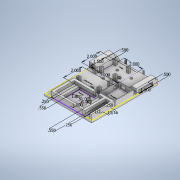
# Autodesk Inventor part: chassis
Saved by Autodesk Inventor 2022 (Build 260153000, 153)
## iProperties
Created: 2021-04-16
Part Number: chassis
Material: Generic
Document SubType Name: Modeling
Designer: kevin
Density: 1 g/cm^3
Appearance: Default
Author: kevin
Autodesk Inventor part; units mm, degrees
ref_plane "YZ Plane" through (0, 0, 0) normal (1, 0, 0) x (0, 1, 0)
ref_plane "XZ Plane" through (0, 0, 0) normal (0, 1, 0) x (-1, 0, 0)
ref_plane "XY Plane" through (0, 0, 0) normal (0, 0, 1) x (1, 0, 0)
sketch "Sketch1" plane through (0, 0, 0) normal (0, 1, 0) x (-1, 0, 0)
  line L0 (63.5, 88.9) -> (-63.5, 88.9)
  line L1 (-63.5, 88.9) -> (-63.5, -88.9)
  line L2 (-63.5, -88.9) -> (63.5, -88.9)
  line L3 (63.5, -88.9) -> (63.5, 88.9)
  line L4 (63.5, 88.9) -> (-63.5, -88.9) construction
  line L5 (-63.5, 88.9) -> (63.5, -88.9) construction
  point P0 (0, 0)
  dimension "d0" = 177.8
  dimension "d1" = 127
  constraints: 12 end point, 2 midpoint, 2 parallel, 1 horizontal, 1 perpendicular
  measures "d0" distance of L2.end L0.start
  measures "d1" distance of L0.start L0.end
extrude "main chassis frame" add sketch "Sketch1" along normal blind 6.35
fillet "chassis front fillet" [suppressed]
fillet "chassis back fillet" [suppressed]
sketch "Sketch3" plane through (63.5, 6.35, 88.9) normal (1, 0, 0) x (0, 0, -1)
  line L0 (0, -6.35) -> (177.8, -6.35) projected
  line L1 (151.8606, -6.35) -> (113.7606, -6.35)
  line L2 (113.7606, -6.35) -> (113.7606, -44.45)
  line L3 (113.7606, -44.45) -> (151.8606, -44.45)
  line L4 (151.8606, -44.45) -> (151.8606, -6.35)
  point P0 (88.9, -6.35)
  point P1 (3.175, -6.35)
  point P2 (174.625, -6.35)
  dimension "d10" = 38.1
  dimension "d11" = 38.1
  constraints: 8 end point, 2 parallel, 1 horizontal, 1 perpendicular, 1 point on line
  measures "d10" distance of L2.end L3.end
  measures "d11" distance of L3.end L1.start
extrude "motor mount" [suppressed]
fillet "round motor mounts" [suppressed]
sketch "Sketch4" plane through (0, 6.35, 0) normal (0, 1, 0) x (1, 0, 0)
  circle A0 centre (15.0812, -75.521) radius 2.3812
  line L0 (15.0812, -75.521) -> (0, -75.521) construction
  circle A1 centre (15.0812, -51.7085) radius 2.3812
  line L1 (15.0812, -51.7085) -> (15.0812, -75.521) construction
  point P0 (0, 0)
  dimension "d15" = 4.7625
  dimension "d17" = 15.0813
  dimension "d19" = 4.7625
  dimension "d20" = 23.8125
  constraints: 4 end point, 2 centre point, 1 horizontal, 1 vertical
  measures "d15" diameter of A0
  measures "d17" distance of L0.start L0.end
  measures "d19" diameter of A1
  measures "d20" distance of L1.start L0.start
extrude "mounting holes for caster" cut sketch "Sketch4" against normal blind 6.35
sketch "Sketch5" plane through (0, 6.35, 0) normal (0, 1, 0) x (1, 0, 0)
  line L0 (63.5, 88.9) -> (-63.5, 88.9) projected
  line L1 (-63.5, -88.9) -> (63.5, -88.9) projected
  line L2 (0, 88.9) -> (-63.5, 88.9)
  line L3 (-63.5, 88.9) -> (-63.5, -88.9)
  line L4 (-63.5, -88.9) -> (0, -88.9)
  line L5 (0, -88.9) -> (0, 88.9)
  point P0 (0, 0)
  point P1 (-63.5, 88.9)
  constraints: 8 end point, 2 parallel, 1 horizontal, 1 midpoint, 1 perpendicular
extrude "cut in half to mirror holes later" cut sketch "Sketch5" against normal blind 6.35
sketch "Sketch6" plane through (0, 0, 0) normal (0, -1, 0) x (1, 0, 0)
  circle A0 centre (19.05, -62.9606) radius 3.175
  line L0 (63.5378, -62.9606) -> (19.0878, -62.9606) construction
  line L1 (19.0878, -62.9606) -> (19.0878, -24.8606) construction
  circle A1 centre (19.05, -24.8606) radius 3.175
  point P0 (0, 0)
  dimension "d26" = 44.45
  dimension "d27" = 6.35
  dimension "d28" = 38.1
  dimension "d29" = 6.35
  constraints: 4 end point, 2 centre point, 1 horizontal, 1 vertical
  measures "d26" distance of L0.start L0.end
  measures "d27" diameter of A0
  measures "d28" distance of L0.end L1.end
  measures "d29" diameter of A1
extrude "zip tie mounting holes for motors" cut sketch "Sketch6" against normal blind 6.35
sketch "Sketch7" plane through (63.5, 6.35, 88.9) normal (1, 0, 0) x (0, 0, -1)
  circle A0 centre (116.9356, -24.2891) radius 1.5875
  line L0 (116.9356, -24.2891) -> (113.7606, -24.2891) construction
  line L1 (113.7606, -30.1625) -> (113.7606, -6.35) projected
  circle A1 centre (148.6856, -24.2891) radius 1.5875
  line L2 (148.6856, -24.2891) -> (151.8606, -24.2891) construction
  line L3 (151.8606, -6.35) -> (151.8606, -30.1625) projected
  point P0 (88.9, -6.35)
  dimension "d32" = 3.175
  dimension "d33" = 3.175
  dimension "d34" = 3.175
  dimension "d35" = 3.175
  constraints: 4 end point, 2 centre point, 2 horizontal, 2 point on line
  measures "d32" distance of L0.start L0.end
  measures "d33" diameter of A0
  measures "d34" diameter of A1
  measures "d35" distance of L2.start L2.end
extrude "motor mount holes" [suppressed]
chamfer "support for motor mounts" [suppressed]
mirror "mirror" about plane through (0, 0, 0) normal (1, 0, 0)
sketch "Sketch8" plane through (0, 6.35, 0) normal (0, 1, 0) x (1, 0, 0)
  circle A0 centre (0, 9.525) radius 6.35
  point P0 (0, 0)
  dimension "d41" = 12.7
  constraints: 1 centre point
  measures "d41" diameter of A0
extrude "hole for motor wires" [suppressed]
sketch "Sketch9" plane through (0, 6.35, 0) normal (0, 1, 0) x (1, 0, 0)
  line L0 (63.5, 76.2) -> (50.8, 76.2)
  line L1 (50.8, 76.2) -> (50.8, 38.1)
  line L2 (50.8, 38.1) -> (63.5, 38.1)
  line L3 (63.5, 38.1) -> (63.5, 76.2)
  line L4 (-39.37, -76.2) -> (-39.37, -26.9875)
  line L5 (-39.37, -26.9875) -> (-25.4, -26.9875)
  line L6 (-25.4, -26.9875) -> (-25.4, -76.2)
  line L7 (-39.37, -26.9875) -> (39.37, -26.9875) construction
  line L8 (39.37, -26.9875) -> (39.37, -33.3375)
  line L9 (39.37, -33.3375) -> (-39.37, -33.3375) construction
  line L10 (-39.37, -33.3375) -> (-39.37, -26.9875)
  line L11 (39.37, -26.9875) -> (25.4, -26.9875)
  line L12 (25.4, -26.9875) -> (25.4, -84.1375)
  line L13 (25.4, -84.1375) -> (39.37, -84.1375)
  line L14 (39.37, -84.1375) -> (39.37, -26.9875)
  line L15 (-25.4, -58.7375) -> (0, -58.7375) construction
  line L16 (0, -58.7375) -> (0, -33.3375) construction
  line L17 (0, -58.7375) -> (25.4, -58.7375) construction
  line L18 (-63.5, -88.9) -> (63.5, -88.9) projected
  line L19 (39.3492, -76.2) -> (39.3492, -88.9)
  line L20 (39.3492, -88.9) -> (-39.37, -88.9)
  line L21 (-39.37, -88.9) -> (-39.37, -76.2)
  line L22 (25.4, -33.3375) -> (12.7, -33.3375) construction
  line L23 (12.7, -33.3375) -> (12.7, -26.9875)
  line L24 (12.7, -26.9875) -> (25.4, -26.9875) construction
  line L25 (25.4, -26.9875) -> (25.4, -33.3375)
  line L26 (12.7, -26.9875) -> (-25.4, -26.9875)
  line L27 (12.7, -33.3375) -> (-25.4, -33.3375)
  line L28 (-39.37, -26.9875) -> (-45.72, -26.9875)
  line L29 (-45.72, -26.9875) -> (-45.72, -88.9)
  line L30 (-45.72, -88.9) -> (-39.37, -88.9)
  line L31 (-39.37, -88.9) -> (-39.37, -26.9875)
  line L32 (-25.4, -33.3375) -> (-39.37, -33.3375)
  line L33 (39.37, -26.9875) -> (45.72, -26.9875)
  line L34 (45.72, -26.9875) -> (45.72, -88.9)
  line L35 (45.72, -88.9) -> (39.37, -88.9)
  line L36 (39.37, -88.9) -> (39.37, -26.9875)
  line L37 (39.37, -33.3375) -> (25.4, -33.3375)
  line L38 (-50.8, 76.2) -> (-63.5, 76.2)
  line L39 (-63.5, 76.2) -> (-63.5, 38.1)
  line L40 (-63.5, 38.1) -> (-50.8, 38.1)
  line L41 (-50.8, 38.1) -> (-50.8, 76.2)
  line L42 (39.37, -84.1375) -> (-39.37, -84.1375)
  line L43 (-39.37, -84.1375) -> (-39.37, -88.9)
  line L44 (-39.37, -88.9) -> (39.37, -88.9)
  line L45 (39.37, -88.9) -> (39.37, -84.1375)
  line L46 (0, -58.7375) -> (0, -84.1375) construction
  line L47 (-25.4, -76.2) -> (-25.4, -84.1375)
  line L48 (-39.37, -88.9) -> (39.37, -88.9)
  line L49 (63.5, -88.9) -> (63.5, 88.9) projected
  line L50 (-63.5, -88.9) -> (-63.5, 88.9) projected
  point P0 (0, 0)
  point P1 (63.5, 85.725)
  point P2 (39.37, -33.3375)
  point P3 (-39.37, -33.3375)
  point P4 (39.3492, -84.1375)
  point P5 (39.37, -84.1375)
  point P6 (39.37, -88.9)
  point P7 (-39.37, -88.9)
  dimension "d45" = 12.7
  dimension "d46" = 13.97
  dimension "d47" = 13.97
  dimension "d48" = 6.35
  dimension "d49" = 25.4
  dimension "d50" = 25.4
  dimension "d51" = 25.4
  dimension "d58" = 6.35
  dimension "d59" = 6.35
  dimension "d65" = 12.7
  dimension "d69" = 25.4
  dimension "d70" = 38.1
  dimension "d71" = 38.1
  constraints: 96 end point, 18 parallel, 11 perpendicular, 11 point on line, 10 horizontal, 5 collinear, 2 midpoint
  measures "d45" distance of L0.start L0.end
  measures "d46" distance of L4.end L5.end
  measures "d47" distance of L7.end L11.end
  measures "d48" distance of L7.end L8.end
  measures "d49" distance of L15.end L16.end
  measures "d50" distance of L15.start L15.end
  measures "d51" distance of L15.end L17.end
  measures "d58" distance of L4.end L28.end
  measures "d59" distance of L7.end L33.end
  measures "d65" distance of L38.start L38.end
  measures "d69" distance of L15.end L46.end
  measures "d70" distance of L0.end L1.end
  measures "d71" distance of L41.start L38.start
extrude "battery walls" add sketch "Sketch9" along normal blind 13.97 contours L21 L18 L29 L28 L4 | L4 L5 L6 L32 | L42 L13 L19 L18 L21 | L6 L26 L23 L27 | L36 L14 L8 L33 L34 L18 | L12 L11 L8 L37
extrude "battery mount underside" add sketch "Sketch9" along normal blind 6.35 contours L4 L32 L6 L47 L42 L21 | L12 L37 L14 L13 | L12 L11 L8 L37
extrude "motor mount spots" [suppressed]
sketch "Sketch12" plane through (0, 6.35, 0) normal (0, 1, 0) x (1, 0, 0)
  line L0 (63.5, 88.9) -> (38.392, 88.9)
  line L1 (38.392, 88.9) -> (38.392, 31.4576)
  line L2 (38.392, 31.4576) -> (63.5, 31.4576)
  line L3 (-38.1, 88.9) -> (-63.5, 88.9)
  line L4 (-63.5, 31.4576) -> (-38.1, 31.4576)
  line L5 (-38.1, 31.4576) -> (-38.1, 88.9)
  line L6 (63.5, 38.1) -> (38.392, 38.1)
  line L7 (38.392, 38.1) -> (38.392, 31.4576)
  line L8 (38.392, 31.4576) -> (63.5, 31.4576)
  line L9 (63.5, 31.4576) -> (63.5, 38.1)
  line L10 (63.5, -88.9) -> (63.5, 88.9) projected
  line L11 (63.5, 76.2) -> (38.392, 76.2)
  line L12 (38.392, 76.2) -> (38.392, 88.9)
  line L13 (38.392, 88.9) -> (63.5, 88.9)
  line L14 (63.5, 88.9) -> (63.5, 76.2)
  line L15 (38.392, 76.2) -> (50.8, 76.2)
  line L16 (50.8, 76.2) -> (50.8, 38.1)
  line L17 (50.8, 38.1) -> (38.392, 38.1)
  line L18 (38.392, 38.1) -> (38.392, 76.2)
  line L19 (-63.5, 38.1) -> (-38.1, 38.1)
  line L20 (-38.1, 38.1) -> (-38.1, 31.4576)
  line L21 (-38.1, 31.4576) -> (-63.5, 31.4576)
  line L22 (-63.5, 31.4576) -> (-63.5, 38.1)
  line L23 (-63.5, -88.9) -> (-63.5, 88.9) projected
  line L24 (-63.5, 76.2) -> (-38.1, 76.2)
  line L25 (-38.1, 76.2) -> (-38.1, 88.9)
  line L26 (-38.1, 88.9) -> (-63.5, 88.9)
  line L27 (-63.5, 88.9) -> (-63.5, 76.2)
  line L28 (-50.8, 76.2) -> (-38.1, 76.2)
  line L29 (-38.1, 76.2) -> (-38.1, 38.1)
  line L30 (-38.1, 38.1) -> (-50.8, 38.1)
  line L31 (-50.8, 38.1) -> (-50.8, 76.2)
  point P0 (0, 0)
  point P1 (63.5, 31.4576)
  point P2 (-63.5, 31.4576)
  constraints: 60 end point, 14 parallel, 8 horizontal, 7 perpendicular, 3 point on line, 1 midpoint
extrude "motor mount covers" add sketch "Sketch12" along normal blind 7.62 contours L10 L11 L1 L0 | L11 L16 L6 L1 | L9 L2 L1 L6 | L5 L24 L23 L3 | L5 L19 L31 L24 | L5 L4 L22 L19
chamfer "motor mount slants" distance 6.35 angle 45 2 edges at (-38.1, 13.97, -60.1788) (38.392, 13.97, -60.1788)
sketch "board placement sketch" plane through (0, 6.35, 0) normal (0, 1, 0) x (1, 0, 0)
  line L0 (-45.72, -26.9875) -> (12.7, -26.9875) projected
  line L1 (12.7, -26.9875) -> (-63.5, -26.9875) construction
  line L2 (-63.5, -26.9875) -> (-63.5, 23.8125) construction
  line L3 (-63.5, 23.8125) -> (12.7, 23.8125) construction
  line L4 (12.7, 23.8125) -> (12.7, -26.9875) construction
  line L5 (12.7, 33.3375) -> (-38.1, 33.3375) construction
  line L6 (-38.1, 33.3375) -> (-38.1, 84.1375) construction
  line L7 (-38.1, 84.1375) -> (12.7, 84.1375) construction
  line L8 (12.7, 84.1375) -> (12.7, 33.3375) construction
  line L9 (58.7375, 19.9847) -> (25.5513, 19.9847) construction
  line L10 (25.5513, 19.9847) -> (25.5513, -23.8125) construction
  line L11 (25.5513, -23.8125) -> (58.7375, -23.8125) construction
  line L12 (58.7375, -23.8125) -> (58.7375, 19.9847) construction
  line L13 (-41.0878, -2.4138) -> (-18.8947, -2.4138) construction
  line L14 (-18.8947, -2.4138) -> (-18.8947, -5.6618) construction
  line L15 (-18.8947, -5.6618) -> (-41.0878, -5.6618) construction
  line L16 (-41.0878, -5.6618) -> (-41.0878, -2.4138) construction
  line L17 (-25.5256, 75.3175) -> (-13.7807, 75.3175) construction
  line L18 (-13.7807, 75.3175) -> (-13.7807, 72.1312) construction
  line L19 (-13.7807, 72.1312) -> (-25.5256, 72.1312) construction
  line L20 (-25.5256, 72.1312) -> (-25.5256, 75.3175) construction
  line L21 (30.9126, -3.1586) -> (52.0855, -3.1586) construction
  line L22 (52.0855, -3.1586) -> (52.0855, -6.4067) construction
  line L23 (52.0855, -6.4067) -> (30.9126, -6.4067) construction
  line L24 (30.9126, -6.4067) -> (30.9126, -3.1586) construction
  line L25 (-19.1836, -39.3523) -> (-6.0554, -39.3523) construction
  line L26 (-6.0554, -39.3523) -> (-6.0554, -43.3784) construction
  line L27 (-6.0554, -43.3784) -> (-19.1836, -43.3784) construction
  line L28 (-19.1836, -43.3784) -> (-19.1836, -39.3523) construction
  line L29 (45.8101, -33.275) -> (58.5101, -33.275) construction
  line L30 (58.5101, -33.275) -> (58.5101, -53.9125) construction
  line L31 (58.5101, -53.9125) -> (45.8101, -53.9125) construction
  line L32 (45.8101, -53.9125) -> (45.8101, -33.275) construction
  line L33 (46.5002, -42.3679) -> (58.1118, -42.3679) construction
  line L34 (58.1118, -42.3679) -> (58.1118, -45.6061) construction
  line L35 (58.1118, -45.6061) -> (46.5002, -45.6061) construction
  line L36 (46.5002, -45.6061) -> (46.5002, -42.3679) construction
  point P0 (0, 0)
  dimension "d85" = 76.2
  dimension "d86" = 50.8
  dimension "d87" = 50.8
  dimension "d88" = 50.8
  dimension "d114" = 20.6375
  dimension "d115" = 12.7
  constraints: 32 end point, 8 parallel, 4 horizontal, 4 perpendicular, 1 point on line, 10 other
  measures "d85" distance of L2.end L3.end
  measures "d86" distance of L3.end L1.start
  measures "d87" distance of L6.end L7.end
  measures "d88" distance of L7.end L5.start
  measures "d114" distance of L29.end L30.end
  measures "d115" distance of L30.end L31.end
sketch "standoff sketch" plane through (0, 6.35, 0) normal (0, 1, 0) x (1, 0, 0)
  line L0 (-38.1, 76.2) -> (-31.75, 76.2)
  line L1 (-31.75, 76.2) -> (-31.75, 69.85)
  line L2 (-31.75, 69.85) -> (-38.1, 69.85)
  line L3 (-38.1, 69.85) -> (-38.1, 76.2)
  line L4 (4.7625, 76.2) -> (-1.5875, 76.2)
  line L5 (-1.5875, 76.2) -> (-1.5875, 69.85)
  line L6 (-1.5875, 69.85) -> (4.7625, 69.85)
  line L7 (4.7625, 69.85) -> (4.7625, 76.2)
  line L8 (-38.1, 33.3375) -> (-31.75, 33.3375)
  line L9 (-31.75, 33.3375) -> (-31.75, 39.6875)
  line L10 (-31.75, 39.6875) -> (-38.1, 39.6875)
  line L11 (-38.1, 39.6875) -> (-38.1, 33.3375)
  line L12 (4.7625, 33.3375) -> (-1.5875, 33.3375)
  line L13 (-1.5875, 33.3375) -> (-1.5875, 39.6875)
  line L14 (-1.5875, 39.6875) -> (4.7625, 39.6875)
  line L15 (4.7625, 39.6875) -> (4.7625, 33.3375)
  circle A0 centre (-34.925, 73.025) radius 1.5875
  circle A1 centre (1.5875, 73.025) radius 1.5875
  circle A2 centre (1.5875, 36.5125) radius 1.5875
  circle A3 centre (-34.925, 36.5125) radius 1.5875
  line L16 (23.7768, -23.8125) -> (22.1893, -23.8125)
  line L17 (22.1893, -23.8125) -> (22.1893, 25.3168)
  line L18 (22.1893, 25.3168) -> (23.7768, 25.3168)
  line L19 (23.7768, 25.3168) -> (23.7768, -23.8125)
  line L20 (22.1893, 25.3168) -> (63.4168, 25.3168)
  line L21 (63.4168, 25.3168) -> (63.4168, 23.7293)
  line L22 (63.4168, 23.7293) -> (22.1893, 23.7293)
  line L23 (22.1893, 23.7293) -> (22.1893, 25.3168)
  line L24 (63.4168, 25.3168) -> (61.8293, 25.3168)
  line L25 (61.8293, 25.3168) -> (61.8293, -25.4)
  line L26 (61.8293, -25.4) -> (63.4168, -25.4)
  line L27 (63.4168, -25.4) -> (63.4168, 25.3168)
  line L28 (63.4168, -25.4) -> (22.1893, -25.4)
  line L29 (22.1893, -25.4) -> (22.1893, -23.8125)
  line L30 (22.1893, -23.8125) -> (63.4168, -23.8125)
  line L31 (63.4168, -23.8125) -> (63.4168, -25.4)
  line L32 (12.7, 17.4692) -> (6.35, 17.4692)
  line L33 (6.35, 17.4692) -> (6.35, 11.1192)
  line L34 (6.35, 11.1192) -> (12.7, 11.1192)
  line L35 (12.7, 11.1192) -> (12.7, 17.4692)
  line L36 (6.35, 17.4692) -> (6.35, 30.1692) construction
  circle A4 centre (9.525, 14.2942) radius 1.5875
  line L37 (6.35, 11.1192) -> (6.35, -11.1058) construction
  line L38 (12.7, -11.1058) -> (6.35, -11.1058)
  line L39 (6.35, -11.1058) -> (6.35, -17.4558)
  line L40 (6.35, -17.4558) -> (12.7, -17.4558)
  line L41 (12.7, -17.4558) -> (12.7, -11.1058)
  circle A5 centre (9.525, -14.2808) radius 1.5875
  line L42 (-46.0375, 30.1625) -> (-39.6875, 30.1625)
  line L43 (-39.6875, 30.1625) -> (-39.6875, 23.8192)
  line L44 (-39.6875, 23.8192) -> (-46.0375, 23.8192)
  line L45 (-46.0375, 23.8192) -> (-46.0375, 30.1625)
  line L46 (-46.0375, 17.4692) -> (-63.5, 17.4692) construction
  line L47 (-63.5, -88.9) -> (-63.5, 88.9) projected
  circle A6 centre (-42.8625, 26.9909) radius 1.5875
  line L48 (-46.0375, -14.2942) -> (-39.6875, -14.2942)
  line L49 (-39.6875, -14.2942) -> (-39.6875, -20.6375)
  line L50 (-39.6875, -20.6375) -> (-46.0375, -20.6375)
  line L51 (-46.0375, -20.6375) -> (-46.0375, -14.2942)
  line L52 (-46.0375, -26.9875) -> (-63.5, -26.9875) construction
  circle A7 centre (-42.8625, -17.4659) radius 1.5875
  line L53 (63.5, -88.9) -> (63.5, 88.9) projected
  line L54 (58.7375, -26.9351) -> (63.5, -26.9351)
  line L55 (63.5, -26.9351) -> (63.5, -88.7773)
  line L56 (63.5, -88.7773) -> (58.7375, -88.7773)
  line L57 (58.7375, -88.7773) -> (58.7375, -26.9351)
  line L58 (45.72, -26.9875) -> (45.72, -88.9) projected
  line L59 (45.72, -26.9875) -> (63.5, -26.9875)
  line L60 (63.5, -26.9875) -> (63.5, -33.3375)
  line L61 (63.5, -33.3375) -> (45.72, -33.3375)
  line L62 (45.72, -33.3375) -> (45.72, -26.9875)
  line L63 (45.72, -60.325) -> (45.72, -53.975)
  line L64 (63.5, -53.975) -> (63.5, -88.7773)
  point P0 (0, 0)
  point P1 (-63.5, 38.1)
  point P2 (63.5, 38.1)
  point P3 (58.7375, -33.3375)
  point P4 (23.7768, 23.7293)
  point P5 (61.8293, 23.7293)
  point P6 (61.8293, -23.8125)
  point P7 (23.7768, -23.8125)
  point P8 (58.7375, -26.9875)
  dimension "d89" = 6.35
  dimension "d90" = 3.175
  dimension "d91" = 1.5875
  dimension "d92" = 1.5875
  dimension "d93" = 1.5875
  dimension "d94" = 1.5875
  dimension "d95" = 12.7
  dimension "d96" = 6.35
  dimension "d97" = 6.35
  dimension "d98" = 3.175
  dimension "d99" = 22.225
  dimension "d100" = 6.35
  dimension "d101" = 6.35
  dimension "d102" = 3.175
  dimension "d106" = 17.4625
  dimension "d107" = 6.35
  dimension "d108" = 6.3433
  dimension "d109" = 3.175
  dimension "d110" = 17.4625
  dimension "d111" = 6.35
  dimension "d112" = 6.3433
  dimension "d113" = 3.175
  dimension "d116" = 4.7625
  dimension "d117" = 6.35
  constraints: 124 end point, 29 parallel, 16 horizontal, 14 perpendicular, 10 point on line, 8 centre point, 1 vertical, 3 other
  measures "d89" distance of L12.end L13.end
  measures "d90" diameter of A2
  measures "d91" distance of L17.end L18.end
  measures "d92" distance of L20.end L21.end
  measures "d93" distance of L25.end L26.end
  measures "d94" distance of L28.end L16.end
  measures "d95" distance of L32.end L36.end
  measures "d96" distance of L32.start L32.end
  measures "d97" distance of L32.end L33.end
  measures "d98" diameter of A4
  measures "d99" distance of L37.end L33.end
  measures "d100" distance of L38.start L37.end
  measures "d101" distance of L37.end L40.start
  measures "d102" diameter of A5
  measures "d106" distance of L46.start L46.end
  measures "d107" distance of L43.end L44.end
  measures "d108" distance of L42.end L43.end
  measures "d109" diameter of A6
  measures "d110" distance of L52.start L52.end
  measures "d111" distance of L49.end L50.end
  measures "d112" distance of L49.start L49.end
  measures "d113" diameter of A7
  measures "d116" distance of L55.end L56.end
  measures "d117" distance of L61.end L58.start
extrude "standoffs" add sketch "standoff sketch" along normal blind 13.97 contours L0 L1 L2 L3 | L7 L6 L5 L4 | L11 L10 L9 L8 | L12 L13 L14 L15 | L30 L25 L28 L29 L16 | L16 L17 L22 L19 | L22 L17 L18 L19 | L19 L20 L25 L22 | L30 L27 L26 L25 | L25 L22 L27 L30 | L25 L20 L21 L22 | L35 L34 L33 L32 | L41 L40 L39 L38 | L42 L43 L44 L45 | L48 L49 L50 L51 | L56 L57 L61 L53 | L61 L57 L59 L53 | L61 L58 L59 L57
sketch "Sketch15" plane through (45.72, 6.35, 33.3375) normal (0, 0, 1) x (1, 0, 0)
  line L0 (-20.32, 0) -> (17.78, 0) projected
  line L1 (13.0175, 0) -> (13.0175, 13.97) projected
  line L2 (0, 0) -> (13.0175, 0)
  line L3 (13.0175, 0) -> (13.0175, 6.35)
  line L4 (13.0175, 6.35) -> (0, 6.35)
  line L5 (0, 6.35) -> (0, 0)
  point P0 (-45.72, -6.35)
  constraints: 8 end point, 2 parallel, 2 point on line, 1 horizontal, 1 perpendicular
extrude "switch wire passage" cut sketch "Sketch15" against normal blind 6.35
sketch "Sketch16" plane through (61.8293, 6.35, 23.8125) normal (0, 0, -1) x (-1, 0, 0)
  line L0 (0, 1.5875) -> (13.0175, 1.5875)
  line L1 (13.0175, 1.5875) -> (13.0175, 9.525)
  line L2 (13.0175, 9.525) -> (0, 9.525)
  line L3 (0, 9.525) -> (0, 1.5875)
  point P0 (61.8293, -6.35)
  constraints: 8 end point, 2 parallel, 1 horizontal, 1 perpendicular
extrude "breadboard to switch wire passage" cut sketch "Sketch16" against normal blind 3.175
sketch "half sonar mount sketch" plane through (63.5, 0, -88.9) normal (0, 0, -1) x (-1, 0, 0)
  line L0 (63.5, 0) -> (88.9, 0)
  line L1 (88.9, 0) -> (88.9, 12.7)
  line L2 (88.9, 12.7) -> (63.5, 12.7)
  line L3 (63.5, 12.7) -> (63.5, 0)
  line L4 (63.5, 12.7) -> (65.0875, 12.7)
  line L5 (65.0875, 0) -> (63.5, 0)
  line L6 (63.5, 0) -> (63.5, 12.7)
  line L7 (88.9, 0) -> (87.3125, 0)
  line L8 (87.3125, 0) -> (87.3125, 12.7)
  line L9 (87.3125, 12.7) -> (88.9, 12.7)
  line L10 (88.9, 12.7) -> (88.9, 0)
  line L11 (87.3125, 0) -> (71.4375, 0)
  line L12 (71.4375, 0) -> (71.4375, 1.5875)
  line L13 (71.4375, 1.5875) -> (87.3125, 1.5875)
  line L14 (87.3125, 1.5875) -> (87.3125, 0)
  line L15 (24.1508, 20.32) -> (102.87, 20.32) projected
  line L16 (63.5104, 20.32) -> (63.5104, -4.1315) construction
  dimension "d130" = 25.4
  dimension "d131" = 12.7
  dimension "d132" = 15.875
  constraints: 32 end point, 7 parallel, 4 horizontal, 3 perpendicular, 1 midpoint, 1 point on line, 1 vertical, 1 other
  measures "d130" distance of L1.end L2.end
  measures "d131" distance of L0.end L1.end
  measures "d132" distance of L12.end L13.end
extrude "half sonar mount" add sketch "half sonar mount sketch" along normal blind 3.175 contours L12 L13 L8 L0 | L8 L2 L1 L0
mirror "sonar mt base mirror" about plane through (0, 0, 0) normal (1, 0, 0) of "half sonar mount"
sketch "Sketch19" plane through (7.9375, 1.5875, -88.9) normal (0, 1, 0) x (1, 0, 0)
  line L0 (15.875, 3.175) -> (0, 3.175) projected
  line L1 (0, 0) -> (0, 3.175) projected
  line L2 (15.875, 3.175) -> (0, 3.175)
  line L3 (0, 3.175) -> (0, 1.5875)
  line L4 (0, 1.5875) -> (15.875, 1.5875)
  line L5 (15.875, 1.5875) -> (15.875, 3.175)
  line L6 (-31.75, 3.175) -> (-15.875, 3.175) projected
  line L7 (-15.875, 3.175) -> (-31.75, 3.175)
  line L8 (-31.75, 3.175) -> (-31.75, 1.5875)
  line L9 (-31.75, 1.5875) -> (-15.875, 1.5875)
  line L10 (-15.875, 1.5875) -> (-15.875, 3.175)
  point P0 (-7.9375, -88.9)
  constraints: 16 end point, 4 parallel, 2 horizontal, 2 perpendicular, 1 midpoint, 1 point on line
extrude "sonar mt buttom" add sketch "Sketch19" along normal blind 1.5875
sketch "Sketch20" plane through (23.8125, 6.35, -88.9) normal (-1, 0, 0) x (0, 0, 1)
  line L0 (-3.175, -3.175) -> (-1.5875, -3.175) projected
  line L1 (0, 6.35) -> (-3.175, 6.35) projected
  line L2 (-3.175, -3.175) -> (-1.5875, -3.175)
  line L3 (-1.5875, -3.175) -> (-1.5875, 6.35)
  line L4 (-1.5875, 6.35) -> (-3.175, 6.35)
  line L5 (-3.175, 6.35) -> (-3.175, -3.175)
  point P0 (88.9, -6.35)
  constraints: 8 end point, 2 parallel, 1 horizontal, 1 midpoint, 1 perpendicular
extrude "sonar mt right" add sketch "Sketch20" along normal blind 1.5875
sketch "Sketch21" plane through (-23.8125, 6.35, -88.9) normal (1, 0, 0) x (0, 0, -1)
  line L0 (3.175, 6.35) -> (3.175, -3.175) projected
  line L1 (0, 6.35) -> (3.175, 6.35) projected
  line L2 (3.175, -3.175) -> (1.5875, -3.175)
  line L3 (1.5875, -3.175) -> (1.5875, 6.35)
  line L4 (1.5875, 6.35) -> (3.175, 6.35)
  line L5 (3.175, 6.35) -> (3.175, -3.175)
  point P0 (-88.9, -6.35)
  constraints: 8 end point, 2 parallel, 1 horizontal, 1 midpoint, 1 perpendicular
extrude "sonar mt left" add sketch "Sketch21" along normal blind 1.5875
sketch "Sketch22" plane through (0, 6.35, 0) normal (0, 1, 0) x (1, 0, 0)
  circle A0 centre (0, 46.0375) radius 6.35
  point P0 (0, 0)
  constraints: 1 centre point
extrude "new hole for motor wires" cut sketch "Sketch22" against normal blind 6.35
sketch "Sketch23" plane through (0, 13.97, 0) normal (0, 1, 0) x (1, 0, 0)
  line L0 (63.5, -88.9) -> (63.5, 88.9) projected
  line L1 (44.742, 31.4576) -> (44.742, 88.9) projected
  line L2 (63.5, 84.1375) -> (44.742, 84.1375)
  line L3 (44.742, 84.1375) -> (44.742, 31.3793)
  line L4 (44.742, 31.3793) -> (63.5, 31.3793)
  line L5 (63.5, 31.3793) -> (63.5, 84.1375)
  line L6 (-44.45, 84.1375) -> (-63.5, 84.1375)
  line L7 (-63.5, 84.1375) -> (-63.5, 31.7464)
  line L8 (-63.5, 31.7464) -> (-44.45, 31.7464)
  line L9 (-44.45, 31.7464) -> (-44.45, 84.1375)
  point P0 (0, 0)
  point P1 (63.5, 31.3793)
  constraints: 16 end point, 4 parallel, 2 horizontal, 2 perpendicular, 2 point on line
extrude "motor mount tops" add sketch "Sketch23" along normal blind 6.35
chamfer "motor mount top slants" distance 6.35 angle 45 2 edges at (-44.45, 20.32, -57.942) (44.742, 20.32, -57.7584)
sketch "Sketch24" plane through (63.4168, 6.35, -25.3168) normal (0, 0, -1) x (-1, 0, 0)
  line L0 (33.3375, 1.5875) -> (22.0251, 1.5875)
  line L1 (22.0251, 1.5875) -> (22.0251, 10.6317)
  line L2 (22.0251, 10.6317) -> (33.3375, 10.6317)
  line L3 (33.3375, 10.6317) -> (33.3375, 1.5875)
  point P0 (63.4168, -6.35)
  constraints: 8 end point, 2 parallel, 1 horizontal, 1 perpendicular
extrude "front passage to breadboard" cut sketch "Sketch24" against normal blind 1.5875
sketch "Sketch25" plane through (23.7768, 6.35, 23.8125) normal (1, 0, 0) x (0, 0, -1)
  line L0 (34.9317, 0) -> (34.9317, 13.97) projected
  line L1 (49.2125, 1.7779) -> (34.9317, 1.7779)
  line L2 (34.9317, 1.7779) -> (34.9317, 9.525)
  line L3 (34.9317, 9.525) -> (49.2125, 9.525)
  line L4 (49.2125, 9.525) -> (49.2125, 1.7779)
  point P0 (23.8125, -6.35)
  constraints: 8 end point, 2 parallel, 1 horizontal, 1 perpendicular, 1 point on line
extrude "another breadboard side access" cut sketch "Sketch25" against normal blind 1.5875
sketch "Sketch26" plane through (0, 6.35, 0) normal (0, 1, 0) x (1, 0, 0)
  line L0 (-45.72, -88.9) -> (-45.72, -26.9875) projected
  line L1 (-45.72, -33.3375) -> (-58.42, -33.3375)
  line L2 (-58.42, -33.3375) -> (-58.42, -53.975)
  line L3 (-58.42, -53.975) -> (-45.72, -53.975)
  line L4 (-45.72, -53.975) -> (-45.72, -33.3375)
  point P0 (0, 0)
  dimension "d152" = 12.7
  dimension "d153" = 20.6375
  constraints: 8 end point, 2 parallel, 1 horizontal, 1 perpendicular, 1 point on line
  measures "d152" distance of L2.end L3.end
  measures "d153" distance of L1.end L2.end
extrude "new switch mount" cut sketch "Sketch26" against normal blind 6.35
sketch "Sketch27" plane through (0, 6.35, 0) normal (0, 1, 0) x (1, 0, 0)
  circle A0 centre (-12.7, -15.875) radius 6.35
  point P0 (0, 0)
  constraints: 1 centre point
extrude "switch wire hole" cut sketch "Sketch27" against normal blind 6.35
body "Solid1"
